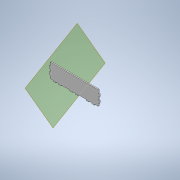
# Autodesk Inventor part: wooden_back
Saved by Autodesk Inventor 2020 (Build 240168000, 168)
## iProperties
Created: 2019-07-24
Part Number: wooden_back
Material: Generic
Document SubType Name: Modeling
Designer: erwin
Density: 1 g/cm^3
Appearance: Default
Author: erwin
Autodesk Inventor part; units mm, degrees
ref_plane "YZ Plane" through (0, 0, 0) normal (1, 0, 0) x (0, 1, 0)
ref_plane "XZ Plane" through (0, 0, 0) normal (0, 1, 0) x (-1, 0, 0)
ref_plane "XY Plane" through (0, 0, 0) normal (0, 0, 1) x (1, 0, 0)
ref_plane "Work Plane1" through (0, 0, 0) normal (0, 0, 1) x (1, 0, 0)
sketch "Sketch1" plane through (0, 0, 0) normal (0, 0, 1) x (1, 0, 0)
  line L0 (0, 72) -> (12, 72)
  line L1 (12, 108) -> (12, 72)
  line L2 (12, 152) -> (12, 108)
  line L3 (0, 152) -> (12, 152)
  line L4 (0, 108) -> (0, 152)
  line L5 (12, 108) -> (0, 108)
  line L6 (0, 72) -> (0, 108)
  line L7 (0, 36) -> (0, 72)
  line L8 (12, 36) -> (0, 36)
  line L9 (12, 36) -> (12, 0)
  line L10 (0, 0) -> (12, 0)
  line L11 (0, -36) -> (0, 0)
  line L12 (12, -36) -> (0, -36)
  line L13 (12, 0) -> (12, -36)
  line L14 (12, 72) -> (12, 36)
  line L15 (0, 0) -> (0, 36)
  line L16 (636, -36) -> (636, -48)
  line L17 (636, -48) -> (588, -48)
  line L18 (588, -48) -> (588, -36)
  line L19 (552, -36) -> (588, -36)
  line L20 (552, -36) -> (552, -48)
  line L21 (552, -48) -> (516, -48)
  line L22 (516, -48) -> (516, -36)
  line L23 (480, -36) -> (516, -36)
  line L24 (480, -36) -> (480, -48)
  line L25 (480, -48) -> (444, -48)
  line L26 (444, -48) -> (444, -36)
  line L27 (408, -36) -> (444, -36)
  line L28 (408, -36) -> (408, -48)
  line L29 (408, -48) -> (372, -48)
  line L30 (372, -48) -> (372, -36)
  line L31 (336, -36) -> (372, -36)
  line L32 (336, -36) -> (336, -48)
  line L33 (336, -48) -> (300, -48)
  line L34 (300, -48) -> (300, -36)
  line L35 (264, -36) -> (300, -36)
  line L36 (264, -36) -> (264, -48)
  line L37 (264, -48) -> (228, -48)
  line L38 (228, -48) -> (228, -36)
  line L39 (192, -36) -> (228, -36)
  line L40 (192, -36) -> (192, -48)
  line L41 (192, -48) -> (156, -48)
  line L42 (156, -48) -> (156, -36)
  line L43 (120, -36) -> (156, -36)
  line L44 (120, -36) -> (120, -48)
  line L45 (120, -48) -> (84, -48)
  line L46 (84, -48) -> (84, -36)
  line L47 (48, -36) -> (84, -36)
  line L48 (48, -36) -> (48, -48)
  line L49 (48, -48) -> (0, -48)
  line L50 (0, -48) -> (0, -36)
  line L51 (0, -36) -> (48, -36)
  line L52 (588, -36) -> (636, -36)
  line L53 (588, -48) -> (552, -48)
  line L54 (516, -36) -> (552, -36)
  line L55 (516, -48) -> (480, -48)
  line L56 (444, -36) -> (480, -36)
  line L57 (444, -48) -> (408, -48)
  line L58 (372, -36) -> (408, -36)
  line L59 (372, -48) -> (336, -48)
  line L60 (300, -36) -> (336, -36)
  line L61 (300, -48) -> (264, -48)
  line L62 (228, -36) -> (264, -36)
  line L63 (228, -48) -> (192, -48)
  line L64 (156, -36) -> (192, -36)
  line L65 (156, -48) -> (120, -48)
  line L66 (84, -36) -> (120, -36)
  line L67 (84, -48) -> (48, -48)
  line L68 (12, 152) -> (636, 152)
  line L69 (636, 152) -> (636, -36)
  line L70 (636, -36) -> (12, -36)
  line L71 (12, -36) -> (12, 152)
  line L72 (324, 152) -> (324, 58) construction
  line L73 (324, 58) -> (636, 58) construction
  line L74 (648, 72) -> (636, 72)
  line L75 (636, 108) -> (636, 72)
  line L76 (636, 152) -> (636, 108)
  line L77 (648, 152) -> (636, 152)
  line L78 (648, 108) -> (648, 152)
  line L79 (636, 108) -> (648, 108)
  line L80 (648, 72) -> (648, 108)
  line L81 (648, 36) -> (648, 72)
  line L82 (636, 36) -> (648, 36)
  line L83 (636, 36) -> (636, 0)
  line L84 (648, 0) -> (636, 0)
  line L85 (648, -36) -> (648, 0)
  line L86 (636, -36) -> (648, -36)
  line L87 (636, 0) -> (636, -36)
  line L88 (636, 72) -> (636, 36)
  line L89 (648, 0) -> (648, 36)
  line L90 (648, -48) -> (648, -36)
  line L91 (636, -36) -> (636, 152)
  line L92 (12, 152) -> (0, 152)
  line L93 (636, 152) -> (636, 164)
  line L94 (636, 164) -> (588, 164)
  line L95 (588, 164) -> (588, 152)
  line L96 (552, 152) -> (588, 152)
  line L97 (552, 152) -> (552, 164)
  line L98 (552, 164) -> (516, 164)
  line L99 (516, 164) -> (516, 152)
  line L100 (480, 152) -> (516, 152)
  line L101 (480, 152) -> (480, 164)
  line L102 (480, 164) -> (444, 164)
  line L103 (444, 164) -> (444, 152)
  line L104 (408, 152) -> (444, 152)
  line L105 (408, 152) -> (408, 164)
  line L106 (408, 164) -> (372, 164)
  line L107 (372, 164) -> (372, 152)
  line L108 (336, 152) -> (372, 152)
  line L109 (336, 152) -> (336, 164)
  line L110 (336, 164) -> (300, 164)
  line L111 (300, 164) -> (300, 152)
  line L112 (264, 152) -> (300, 152)
  line L113 (264, 152) -> (264, 164)
  line L114 (264, 164) -> (228, 164)
  line L115 (228, 164) -> (228, 152)
  line L116 (192, 152) -> (228, 152)
  line L117 (192, 152) -> (192, 164)
  line L118 (192, 164) -> (156, 164)
  line L119 (156, 164) -> (156, 152)
  line L120 (120, 152) -> (156, 152)
  line L121 (120, 152) -> (120, 164)
  line L122 (120, 164) -> (84, 164)
  line L123 (84, 164) -> (84, 152)
  line L124 (48, 152) -> (84, 152)
  line L125 (48, 152) -> (48, 164)
  line L126 (48, 164) -> (0, 164)
  line L127 (0, 164) -> (0, 152)
  line L128 (0, 152) -> (48, 152)
  line L129 (588, 152) -> (636, 152)
  line L130 (588, 164) -> (552, 164)
  line L131 (516, 152) -> (552, 152)
  line L132 (516, 164) -> (480, 164)
  line L133 (444, 152) -> (480, 152)
  line L134 (444, 164) -> (408, 164)
  line L135 (372, 152) -> (408, 152)
  line L136 (372, 164) -> (336, 164)
  line L137 (300, 152) -> (336, 152)
  line L138 (300, 164) -> (264, 164)
  line L139 (228, 152) -> (264, 152)
  line L140 (228, 164) -> (192, 164)
  line L141 (156, 152) -> (192, 152)
  line L142 (156, 164) -> (120, 164)
  line L143 (84, 152) -> (120, 152)
  line L144 (84, 164) -> (48, 164)
  line L145 (636, 152) -> (12, 152)
  line L146 (636, 152) -> (648, 152)
  line L147 (648, 164) -> (648, 152)
  constraints: 296 end point, 53 symmetric about line, 41 horizontal, 28 vertical, 3 perpendicular, 2 midpoint, 2 parallel, 46 other
extrude "Extrusion1" add sketch "Sketch1" along normal blind 12 contours L6 L5 L1 L0 | L1 L2 L68 L69 L52 L19 L54 L23 L56 L27 L58 L31 L60 L35 L62 L39 L64 L43 L66 L47 L51 L13 L9 L14 | L8 L9 L10 L15 | L47 L46 L67 L48 | L43 L42 L65 L44 | L35 L34 L61 L36 | L31 L30 L59 L32 | L23 L22 L55 L24 | L19 L18 L53 L20 | L79 L80 L74 L69 | L69 L82 L89 L84
ref_plane "Work Plane2" through (0, -113.0256, -190.9643) normal (-1, 0, 0) x (0, -0.5, 0.8660254)
ref_plane "Work Plane3" through (0, -113.0256, -190.9643) normal (-1, 0, 0) x (0, -0.5, 0.8660254)
body "Solid1"
